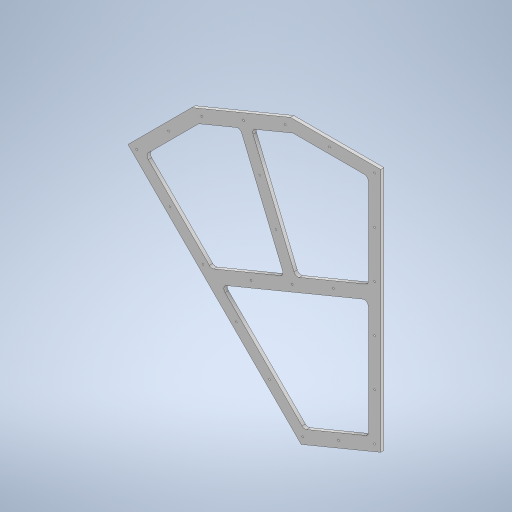
# Autodesk Inventor part: ДМС 206 Крепление сетки к кассете
Saved by Autodesk Inventor 2024.2 (Build 282272000, 272)
## iProperties
Created: 2024-05-05
Part Number: ДМС 206 Крепление сетки к кассете
Material: Generic
Document SubType Name: Modeling
Designer: pokla
Density: 1 g/cm^3
Appearance: Default
Author: pokla
Autodesk Inventor part; units mm, degrees
ref_plane "YZ Plane" through (0, 0, 0) normal (1, 0, 0) x (0, 1, 0)
ref_plane "XZ Plane" through (0, 0, 0) normal (0, 1, 0) x (-1, 0, 0)
ref_plane "XY Plane" through (0, 0, 0) normal (0, 0, 1) x (1, 0, 0)
sketch "Sketch1" plane through (0, 0, 0) normal (0, 0, 1) x (1, 0, 0)
  line L0 (0, 273.8452) -> (193.6378, 193.6378) construction
  line L1 (193.6378, 193.6378) -> (273.8452, 0) construction
  line L2 (273.8452, 0) -> (193.6378, -193.6378) construction
  line L3 (193.6378, -193.6378) -> (0, -273.8452) construction
  line L4 (0, -273.8452) -> (-193.6378, -193.6378) construction
  line L5 (-193.6378, -193.6378) -> (-273.8452, 0) construction
  line L6 (-273.8452, 0) -> (-193.6378, 193.6378) construction
  line L7 (-193.6378, 193.6378) -> (0, 273.8452)
  line L8 (-193.6378, 193.6378) -> (0, 273.8452)
  line L9 (-459.9272, 770.6562) -> (-219.7185, 870.1539)
  line L10 (-96.8189, 233.7415) -> (-339.8229, 820.405) construction
  line L11 (-219.7185, 870.1539) -> (0, 870.1539)
  line L12 (0, 870.1539) -> (0, 273.8452)
  line L13 (-459.9272, 770.6562) -> (-615.2917, 615.2917)
  line L14 (-615.2917, 615.2917) -> (-193.6378, 193.6378)
  point P0 (0, 0)
  point P1 (0, 0)
  dimension "d0" = 506
  dimension "d2" = 260
  dimension "d3" = 635
  constraints: 30 end point, 2 midpoint, 1 coincident, 1 horizontal, 1 parallel, 1 perpendicular, 1 symmetric about line, 1 vertical, 1 vertical alignment, 17 other
  measures "d0" distance between parallel lines of L5 L1
  measures "d2" distance of L9.start L9.end
  measures "d3" distance of L10.end L10.start
extrude "Extrusion1" add sketch "Sketch1" along normal mid plane 8
sketch "Sketch2" plane through (0, 0, 4) normal (0, 0, 1) x (1, 0, 0)
  line L0 (-219.7185, 870.1539) -> (-459.9272, 770.6562) projected
  line L1 (-459.9272, 770.6562) -> (-615.2917, 615.2917) projected
  line L2 (-235.0492, 528.2621) -> (-412.382, 454.8085)
  line L3 (-193.6378, 193.6378) -> (0, 273.8452) projected
  line L4 (-96.8189, 233.7415) -> (-339.8229, 820.405) construction
  line L5 (-615.2917, 615.2917) -> (-193.6378, 193.6378) projected
  line L6 (-412.382, 454.8085) -> (-572.8653, 615.2917)
  line L7 (-572.8653, 615.2917) -> (-442.9336, 745.2234)
  line L8 (-442.9336, 745.2234) -> (-342.2006, 786.9484)
  line L9 (-235.0492, 528.2621) -> (-342.2006, 786.9484)
  line L10 (-207.3328, 539.7426) -> (-30, 613.1963)
  line L11 (-30, 613.1963) -> (-30, 840.1539)
  line L12 (-30, 840.1539) -> (-213.7512, 840.1539)
  line L13 (-213.7512, 840.1539) -> (-314.4842, 798.4289)
  line L14 (-207.3328, 539.7426) -> (-314.4842, 798.4289)
  line L15 (0, 273.8452) -> (0, 870.1539) projected
  line L16 (-412.382, 454.8085) -> (-30, 613.1963) construction
  line L17 (-389.421, 431.8474) -> (-30, 580.7245)
  line L18 (-186.5988, 229.0252) -> (-30, 293.8906)
  line L19 (-30, 293.8906) -> (-30, 580.7245)
  line L20 (-186.5988, 229.0252) -> (-389.421, 431.8474)
  point P0 (0, 0)
  dimension "d11" = 30
  dimension "d12" = 280
  dimension "d13" = 30
  dimension "d14" = 30
  dimension "d15" = 15
  dimension "d21" = 30
  dimension "d22" = 30
  dimension "d23" = 30
  dimension "d24" = 30
  constraints: 32 end point, 5 parallel, 5 symmetric about line, 2 midpoint, 1 collinear
  measures "d11" distance between parallel lines of L5 L6
  measures "d12" distance between parallel lines of L8 L2
  measures "d13" distance between parallel lines of L0 L8
  measures "d14" distance between parallel lines of L1 L7
  measures "d15" distance between parallel lines of L9 L4
  measures "d21" distance between parallel lines of L16 L17
  measures "d22" distance between parallel lines of L5 L20
  measures "d23" distance between parallel lines of L19 L15
  measures "d24" distance between parallel lines of L18 L3
extrude "Extrusion2" cut sketch "Sketch2" against normal up to surface (8 mm away)
fillet "Fillet1" radius 10 12 edges at (-572.8653, 615.2917, 0) (-342.2006, 786.9484, 0) (-235.0492, 528.2621, 0) (-412.382, 454.8085, 0) (-314.4842, 798.4289, 0) (-30, 840.1539, 0) (-30, 613.1963, 0) (-207.3328, 539.7426, 0) (-389.421, 431.8474, 0) (-30, 580.7245, 0) (-30, 293.8906, 0) (-186.5988, 229.0252, 0)
sketch "Sketch5" plane through (0, 0, 4) normal (0, 0, 1) x (1, 0, 0)
  line L0 (-219.7185, 870.1539) -> (-459.9272, 770.6562) projected
  line L1 (0, 870.1539) -> (-219.7185, 870.1539) projected
  line L2 (-459.9272, 770.6562) -> (-615.2917, 615.2917) projected
  line L3 (-615.2917, 615.2917) -> (-193.6378, 193.6378) projected
  line L4 (-193.6378, 193.6378) -> (0, 273.8452) projected
  line L5 (0, 273.8452) -> (0, 870.1539) projected
  line L6 (-15, 855.1539) -> (-216.7349, 855.1539) construction
  line L7 (-216.7349, 855.1539) -> (-451.4304, 757.9398) construction
  line L8 (-451.4304, 757.9398) -> (-594.0785, 615.2917) construction
  line L9 (-594.0785, 615.2917) -> (-190.1183, 211.3315) construction
  line L10 (-190.1183, 211.3315) -> (-15, 283.8679) construction
  line L11 (-15, 283.8679) -> (-15, 855.1539) construction
  line L12 (-375.5942, 437.5747) -> (-43.8268, 574.9973) projected
  line L13 (-211.1597, 548.9814) -> (-310.6574, 789.1901) projected
  line L14 (-415.9015, 437.1147) -> (-15, 603.1736) construction
  line L15 (-215.4508, 520.1442) -> (-334.0826, 806.5468) construction
  circle A0 centre (-334.0826, 806.5468) radius 2
  circle A1 centre (-215.4508, 520.1442) radius 2
  circle A2 centre (-294.54, 711.0824) radius 2
  circle A3 centre (-254.9973, 615.6179) radius 2
  circle A4 centre (-594.0785, 615.2917) radius 2
  circle A5 centre (-513.2865, 534.4997) radius 2
  circle A6 centre (-432.4944, 453.7076) radius 2
  circle A7 centre (-351.7024, 372.9156) radius 2
  circle A8 centre (-270.9103, 292.1235) radius 2
  circle A9 centre (-190.1183, 211.3315) radius 2
  circle A10 centre (-315.6917, 478.623) radius 2
  circle A11 centre (-102.5592, 247.5997) radius 2
  circle A12 centre (-516.2968, 693.0734) radius 2
  circle A13 centre (-435.7094, 764.4517) radius 2
  circle A14 centre (-15, 855.1539) radius 2
  circle A15 centre (-15, 740.8967) radius 2
  circle A16 centre (-15, 626.6395) radius 2
  circle A17 centre (-15, 512.3823) radius 2
  circle A18 centre (-15, 398.1251) radius 2
  circle A19 centre (-15, 283.8679) radius 2
  circle A20 centre (-115.2098, 561.6653) radius 2
  circle A21 centre (-125, 855.1539) radius 2
  circle A22 centre (-232.4559, 848.642) radius 2
  point P0 (0, 0)
  dimension "d32" = 15
  dimension "d33" = 15
  dimension "d34" = 15
  dimension "d35" = 4
  dimension "d37" = 103.33
  dimension "d38" = 103.33
  dimension "d43" = 114.2572
  dimension "d49" = 108.5
  dimension "d50" = 110
  dimension "d51" = 110
  constraints: 23 centre point, 16 end point, 9 symmetric about line, 8 equal radius, 7 point on line, 3 coincident, 3 midpoint, 2 parallel, 25 other
  measures "d32" distance between parallel lines of L5 L11
  measures "d33" distance between parallel lines of L12 L14
  measures "d34" distance between parallel lines of L13 L15
  measures "d35" diameter of A0
  measures "d37" distance of A2.centre A0.centre
  measures "d38" distance of A3.centre A2.centre
  measures "d43" distance of A4.centre A5.centre
  measures "d49" distance of A1.centre A10.centre
  measures "d50" distance of A12.centre A4.centre
  measures "d51" distance of A13.centre A0.centre
extrude "Extrusion4" cut sketch "Sketch5" against normal up to surface (8 mm away) contours A0 | A1 | A2 | A3 | A4 | A5 | A6 | A7 | A8 | A9 | A10 | A11 | A12 | A13 | A14 | A15 | A16 | A17 | A18 | A19 | A20 | A21 | A22
equation "\"d0\" = Барабан_габарит_по_кассетам"
equation "\"d2\" = Кассета_длина_грани"
equation "\"d3\" = Кассета_высота"
equation "\"d11\" = d13"
equation "\"d14\" = d13"
equation "\"d15\" = 0.5 * d13"
equation "\"d21\" = d13"
equation "\"d22\" = d13"
equation "\"d23\" = d13"
equation "\"d24\" = d13"
equation "\"Барабан_габарит_по_кассетам\" = 506"
equation "\"Кассета_длина_грани\" = 260"
equation "\"Кассета_высота\" = 635"
body "Solid1"
